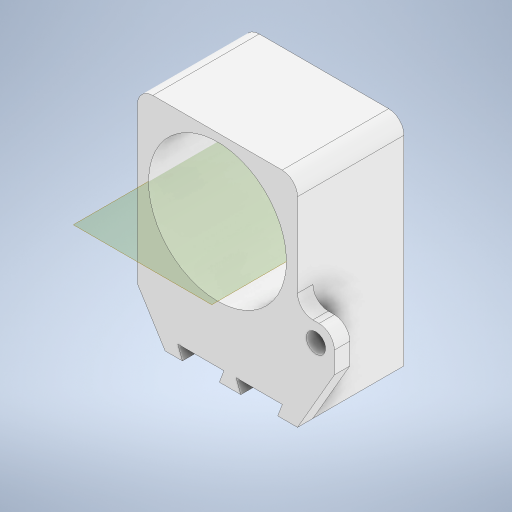
# Autodesk Inventor part: Brushless Motor Seat
Saved by Autodesk Inventor 2024 (Build 280153000, 153)
## iProperties
Created: 2023-11-02
Part Number: Brushless Motor Seat
Material: Generic
Document SubType Name: Modeling
Designer: CJ110
Density: 1 g/cm^3
Appearance: Default
Author: CJ110
## iProperties of the stored document Brushless Motor Seat_3DPrint.ipt
Created: 2023-11-03
Part Number: Brushless Motor Seat_3DPrint
Material: Generic
Document SubType Name: Modeling
Designer: CJ110
Density: 1 g/cm^3
Appearance: Default
Author: CJ110
Autodesk Inventor part; units mm, degrees
ref_plane "YZ Plane" through (0, 0, 0) normal (1, 0, 0) x (0, 1, 0)
ref_plane "XZ Plane" through (0, 0, 0) normal (0, 1, 0) x (-1, 0, 0)
ref_plane "XY Plane" through (0, 0, 0) normal (0, 0, 1) x (1, 0, 0)
ref_plane "Work Plane1" through (-2.4672, -28.2462, -31.996) normal (1, 0, 0) x (0, 1, 0)
sketch "Sketch1" plane through (-2.4672, -28.2462, -31.996) normal (1, 0, 0) x (0, 1, 0)
  line L0 (0, 16.54) -> (22, 16.54)
  line L1 (22, 16.54) -> (22, -16.54)
  line L2 (22, -16.54) -> (0, -16.54)
  line L3 (0, -16.54) -> (0, 16.54)
  line L4 (0, -14) -> (0, 14) projected
  line L5 (0, 13) -> (22, 13) construction
  line L6 (0, -13) -> (22, -13) construction
  line L7 (22, -14) -> (22, 14) projected
  line L8 (22, 0) -> (0, 0) construction
  point P0 (28.2462, 31.996)
  dimension "d3" = 33.08
  constraints: 14 end point, 4 horizontal, 2 collinear, 2 midpoint, 2 parallel, 1 perpendicular, 2 other
  measures "d3" distance of L2.end L0.start
extrude "Extrusion1" add sketch "Sketch1" along normal blind 28.575 and the other way blind 15.875
sketch "Sketch5" plane through (-18.3422, -6.2462, -15.456) normal (0, 1, 0) x (1, 0, 0)
  circle A0 centre (15.875, 16.54) radius 4.5 projected
  circle A1 centre (15.875, 16.54) radius 14 projected
  circle A2 centre (15.875, 16.54) radius 14.254
  point P0 (18.3422, -15.456)
  dimension "d9" = 0.254
  constraints: 1 centre point
  measures "d9" radial gap between concentric circles of A1 A2
extrude "Extrusion2" cut sketch "Sketch5" against normal through all contours A0 | A1 | A2
sketch "Sketch6" plane through (-18.3422, -6.2462, -15.456) normal (0, 1, 0) x (1, 0, 0)
  circle A0 centre (15.875, 16.54) radius 14.254 projected
  line L0 (0, 0) -> (44.45, 0) projected
  line L1 (44.45, 33.08) -> (44.45, 0) projected
  line L2 (0, 33.08) -> (44.45, 33.08) projected
  line L3 (0, 0) -> (0, 33.08) projected
  line L4 (44.45, 9.301) -> (41.91, 8.3485)
  line L5 (41.91, 8.3485) -> (41.91, 17.8735)
  line L6 (41.91, 17.8735) -> (44.45, 16.921)
  line L7 (44.45, 21.366) -> (41.91, 20.4135)
  line L8 (41.91, 20.4135) -> (41.91, 29.9385)
  line L9 (41.91, 29.9385) -> (44.45, 28.986)
  line L10 (0, 0) -> (0, 33.08) projected
  line L11 (0, 16.54) -> (44.6434, 16.54) construction
  point P0 (18.3422, -15.456)
  point P1 (41.91, 25.176)
  point P2 (41.91, 13.111)
  dimension "d12" = 9.525
  dimension "d13" = 7.62
  dimension "d14" = 7.62
  dimension "d15" = 2.54
  dimension "d61" = 8.636
  dimension "d62" = 12.065
  constraints: 14 end point, 5 point on line, 4 equal length, 3 midpoint, 2 vertical, 1 perpendicular
  measures "d12" distance of L4.end L5.end
  measures "d13" distance of L4.start L6.end
  measures "d14" distance of L9.end L7.start
  measures "d15" distance between parallel lines of L1 L5
  measures "d61" distance from line of point (41.91, 25.176) L11
  measures "d62" distance of point (41.91, 25.176) point (41.91, 13.111)
extrude "Extrusion3" cut sketch "Sketch6" against normal through all contours L4 L5 L6 L1 | L1 L7 L8 L9
sketch "Sketch7" plane through (-18.3422, -28.2462, -15.456) normal (0, -1, 0) x (1, 0, 0)
  circle A0 centre (4.335, -28.08) radius 1.524 projected
  circle A1 centre (4.335, -5) radius 1.524 projected
  circle A2 centre (27.415, -5) radius 1.524 projected
  circle A3 centre (27.415, -28.08) radius 1.524 projected
  line L0 (3.2574, -29.1576) -> (2.1797, -28.08)
  line L1 (2.1797, -28.08) -> (3.2574, -27.0024)
  line L2 (44.45, -28.986) -> (41.91, -29.9385) projected
  line L3 (41.91, -29.9385) -> (41.91, -20.4135) projected
  line L4 (41.91, -20.4135) -> (44.45, -21.366) projected
  line L5 (44.45, -16.921) -> (44.45, -21.366) projected
  line L6 (44.45, -16.921) -> (41.91, -17.8735) projected
  line L7 (41.91, -17.8735) -> (41.91, -8.3485) projected
  line L8 (41.91, -8.3485) -> (44.45, -9.301) projected
  line L9 (44.45, 0) -> (44.45, -9.301) projected
  line L10 (44.45, 0) -> (0, 0) projected
  line L11 (0, -33.08) -> (0, 0) projected
  line L12 (0, -33.08) -> (44.45, -33.08) projected
  line L13 (44.45, -28.986) -> (44.45, -33.08) projected
  circle A4 centre (15.875, -16.54) radius 14.254 projected
  line L14 (3.2574, -6.0776) -> (2.1797, -5)
  line L15 (2.1797, -5) -> (3.2574, -3.9224)
  line L16 (26.3374, -6.0776) -> (25.2597, -5)
  line L17 (25.2597, -5) -> (26.3374, -3.9224)
  line L18 (26.3374, -29.1576) -> (25.2597, -28.08)
  line L19 (25.2597, -28.08) -> (26.3374, -27.0024)
  point P0 (18.3422, 15.456)
  constraints: 16 end point, 8 point on circle, 8 tangent, 4 horizontal alignment, 4 perpendicular
extrude "Extrusion4" cut sketch "Sketch7" against normal blind 3.175 contours A0 | A0 L0 L1 | A1 | A1 L14 L15 | A2 | A2 L16 L17 | A3 | A3 L18 L19
fillet "Fillet1" radius 3.175 2 edges at (-18.3422, -17.2462, -48.536) (-18.3422, -17.2462, -15.456)
sketch "Sketch8" plane through (23.5678, -6.2462, -23.8045) normal (0, 1, 0) x (1, 0, 0)
  line L0 (5.715, -17.081) -> (5.715, -4.381)
  line L1 (5.715, -4.381) -> (-14.605, -17.081) construction
  line L2 (-14.605, -17.081) -> (5.715, -17.081)
  line L3 (-38.735, -8.3485) -> (2.54, -8.3485) projected
  line L4 (2.54, 0.9525) -> (2.54, -8.3485) projected
  line L5 (-16.2877, -14.3886) -> (4.0323, -1.6886)
  line L6 (-14.605, -17.081) -> (-16.2877, -14.3886)
  line L7 (5.715, -4.381) -> (4.0323, -1.6886)
  dimension "d26" = 20.32
  dimension "d27" = 12.7
  dimension "d28" = 8.7325
  dimension "d29" = 3.175
  dimension "d30" = 3.175
  constraints: 12 end point, 3 perpendicular, 1 parallel, 1 vertical
  measures "d26" distance of L1.end L0.start
  measures "d27" distance of L0.start L0.end
  measures "d28" distance from line of L3 L1.end
  measures "d29" distance from line of L4 L0.end
  measures "d30" distance between parallel lines of L1 L5
extrude "Extrusion5" cut sketch "Sketch8" along normal through all both and the other way through all
sketch "Sketch11" plane through (23.5678, -6.2462, -23.8045) normal (0, 1, 0) x (1, 0, 0)
  line L0 (2.54, 20.6375) -> (2.54, 24.7315) projected
  line L1 (2.54, 24.7315) -> (-10.6582, 32.3515)
  line L2 (-10.6582, 32.3515) -> (-18.2782, 32.3515)
  line L3 (-18.2782, 32.3515) -> (-18.2782, 24.7315)
  circle A0 centre (-26.035, 8.1915) radius 14.254 projected
  line L4 (-6.6235, -8.3485) -> (2.54, -2.6213) projected
  line L5 (2.54, 0.9525) -> (2.54, -2.6213) projected
  line L6 (2.54, 0.9525) -> (0, 0) projected
  line L7 (0, 0) -> (0, 9.525) projected
  line L8 (0, 9.525) -> (2.54, 8.5725) projected
  line L9 (2.54, 13.0175) -> (2.54, 8.5725) projected
  line L10 (2.54, 13.0175) -> (0, 12.065) projected
  line L11 (0, 12.065) -> (0, 21.59) projected
  line L12 (0, 21.59) -> (2.54, 20.6375) projected
  line L13 (2.54, 24.7315) -> (2.54, 20.6375) projected
  line L14 (-38.735, 24.7315) -> (2.54, 24.7315) projected
  arc A1 (-38.735, 24.7315) -> (-41.91, 21.5565) centre (-38.735, 21.5565) ccw projected
  line L15 (-41.91, -5.1735) -> (-41.91, 21.5565) projected
  arc A2 (-41.91, -5.1735) -> (-38.735, -8.3485) centre (-38.735, -5.1735) ccw projected
  line L16 (-38.735, -8.3485) -> (-6.6235, -8.3485) projected
  circle A3 centre (-14.4682, 28.5415) radius 1.5875
  point P0 (-23.5678, -23.8045)
  point P1 (2.54, 24.7315)
  point P2 (-41.91, 8.1915)
  dimension "d42" = 120
  dimension "d43" = 7.62
  dimension "d45" = 7.62
  dimension "d46" = 3.175
  dimension "d47" = 3.81
  dimension "d48" = 3.81
  dimension "d53" = 20.35
  dimension "d63" = 11.5668
  constraints: 6 end point, 2 perpendicular, 1 centre point, 1 midpoint, 1 point on line
  measures "d42" angle of L0 L1
  measures "d43" distance between parallel lines of L14 L2
  measures "d45" distance of L1.end L2.end
  measures "d46" diameter of A3
  measures "d47" distance from line of L3 A3.centre
  measures "d48" distance from line of L2 A3.centre
  measures "d53" vertical distance of A3.centre point (-41.91, 8.191)
  measures "d63" horizontal distance of A3.centre A0.centre
extrude "Extrusion7" add sketch "Sketch11" against normal blind 3.175 contours L14 L3 L2 L1 | A3
fillet "Fillet2" radius 3.175 1 edges at (5.2896, -7.8337, -56.156)
fillet "Fillet3" radius 3.175 1 edges at (5.2896, -7.8337, -48.536)
hole "Hole2" at (9.0996, -6.2462, -52.346) direction (0, -1, 0) diameter 4 depth 3.175 clearance for "Hex Head Machine Screw" size "M4" standard "Ansi Metric M Profile"
equation "\"d45\" = d43"
equation "\"d47\" = 0.5 * d43"
equation "\"d48\" = 0.5 * d43"
body "Solid1"
